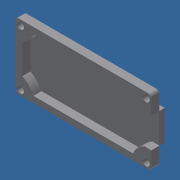
# Autodesk Inventor part: contramoldetapasevo
Saved by Autodesk Inventor 2014 (Build 180170000, 170)
## iProperties
Created: 2014-04-18
Part Number: contramoldetapasevo
Material: Generic
Document SubType Name: Modeling
Designer: Lefo
Density: 1 g/cm^3
Appearance: Default
Author: Lefo
Autodesk Inventor part; units mm, degrees
ref_plane "YZ Plane" through (0, 0, 0) normal (1, 0, 0) x (0, 1, 0)
ref_plane "XZ Plane" through (0, 0, 0) normal (0, 1, 0) x (-1, 0, 0)
sketch "Sketch1" plane through (0, 0, 0) normal (0, 0, 1) x (1, 0, 0)
  line L0 (17.4, 4.3375) -> (19.4, 4.3375) projected
  line L1 (19.4, 8.4) -> (19.4, 4.3375) projected
  arc A0 (19.4, 8.4) -> (18.4, 9.4) centre (18.4, 8.4) ccw projected
  line L2 (-18.4, 9.4) -> (18.4, 9.4) projected
  arc A1 (-18.4, 9.4) -> (-19.4, 8.4) centre (-18.4, 8.4) ccw projected
  line L3 (-19.4, -8.4) -> (-19.4, 8.4) projected
  arc A2 (-19.4, -8.4) -> (-18.4, -9.4) centre (-18.4, -8.4) ccw projected
  line L4 (18.4, -9.4) -> (-18.4, -9.4) projected
  arc A3 (18.4, -9.4) -> (19.4, -8.4) centre (18.4, -8.4) ccw projected
  line L5 (19.4, -4.2375) -> (19.4, -8.4) projected
  line L6 (19.4, -4.2375) -> (17.4, -4.2375) projected
  arc A4 (17.4, -4.2375) -> (14.1485, -7.6) centre (20.15, -10.15) ccw projected
  line L7 (14.1485, -7.6) -> (-14.247, -7.6) projected
  arc A5 (-14.247, -7.6) -> (-17.4, -4.3375) centre (-20.15, -10.15) ccw projected
  line L8 (-17.4, -4.3375) -> (-17.4, 4.2375) projected
  arc A6 (-17.4, 4.2375) -> (-14.1485, 7.6) centre (-20.15, 10.15) ccw projected
  line L9 (-14.1485, 7.6) -> (14.247, 7.6) projected
  arc A7 (14.247, 7.6) -> (17.4, 4.3375) centre (20.15, 10.15) ccw projected
  circle A8 centre (-17.9, -7.9) radius 1 projected
  circle A9 centre (17.9, -7.9) radius 1 projected
  circle A10 centre (-17.9, 7.9) radius 1 projected
  circle A11 centre (17.9, 7.9) radius 1 projected
  line L10 (19.4, -2.5) -> (19.4, 2.5) projected
  line L11 (19.4, 8.4) -> (19.4, 2.5) projected
  line L12 (19.4, -2.5) -> (19.4, -8.4) projected
  point P0 (0, 0)
ref_plane "Work Plane1" through (-26.7016, -22.7609, 2.3) normal (0, 0, 1) x (1, 0, 0)
extrude "Extrusion1" add sketch "Sketch1" along normal up to surface (2.3 mm away) contours A7 L9 A6 L8 A5 L7 A4 L6 L5 A3 L4 A2 L3 A1 L2 A0 L1 L0
sketch "Sketch2" plane through (0, 0, 0) normal (0, 0, -1) x (-1, 0, 0)
  arc A0 (14.1485, 7.6) -> (17.4, 4.2375) centre (20.15, 10.15) ccw projected
  line L0 (17.4, -4.3375) -> (17.4, 4.2375) projected
  arc A1 (17.4, -4.3375) -> (14.247, -7.6) centre (20.15, -10.15) ccw projected
  line L1 (-14.1485, -7.6) -> (14.247, -7.6) projected
  arc A2 (-14.1485, -7.6) -> (-17.4, -4.2375) centre (-20.15, -10.15) ccw projected
  line L2 (-17.4, -4.2375) -> (-19.4, -4.2375) projected
  line L3 (-19.4, -4.2375) -> (-19.4, 4.3375) projected
  line L4 (-19.4, 4.3375) -> (-17.4, 4.3375) projected
  arc A3 (-17.4, 4.3375) -> (-14.247, 7.6) centre (-20.15, 10.15) ccw projected
  line L5 (14.1485, 7.6) -> (-14.247, 7.6) projected
  point P0 (0, 0)
extrude "Extrusion2" add sketch "Sketch2" along normal blind 1.5
sketch "Sketch3" plane through (0, 0, 0) normal (0, 0, 1) x (1, 0, 0)
  line L0 (19.4, 4.3375) -> (19.4, -4.2375) projected
  line L1 (17.4, 4.3375) -> (19.4, 4.3375) projected
  arc A0 (14.247, 7.6) -> (17.4, 4.3375) centre (20.15, 10.15) ccw projected
  line L2 (-14.1485, 7.6) -> (14.247, 7.6) projected
  arc A1 (-17.4, 4.2375) -> (-14.1485, 7.6) centre (-20.15, 10.15) ccw projected
  line L3 (-17.4, -4.3375) -> (-17.4, 4.2375) projected
  arc A2 (-14.247, -7.6) -> (-17.4, -4.3375) centre (-20.15, -10.15) ccw projected
  line L4 (14.1485, -7.6) -> (-14.247, -7.6) projected
  arc A3 (17.4, -4.2375) -> (14.1485, -7.6) centre (20.15, -10.15) ccw projected
  line L5 (19.4, -4.2375) -> (17.4, -4.2375) projected
  arc A4 (13.332, 6.1) -> (17.0815, 2.8375) centre (20.15, 10.15) ccw
  line L6 (17.0815, 2.8375) -> (17.9, 2.8375)
  line L7 (17.9, 2.8375) -> (17.9, -2.7375)
  line L8 (17.9, -2.7375) -> (17.0861, -2.7375)
  arc A5 (17.0861, -2.7375) -> (13.2269, -6.1) centre (20.15, -10.15) ccw
  line L9 (13.2269, -6.1) -> (-13.332, -6.1)
  arc A6 (-13.332, -6.1) -> (-15.9, -3.4548) centre (-20.15, -10.15) ccw
  line L10 (-15.9, -3.4548) -> (-15.9, 3.3478)
  arc A7 (-15.9, 3.3478) -> (-13.2269, 6.1) centre (-20.15, 10.15) ccw
  line L11 (-13.2269, 6.1) -> (13.332, 6.1)
  line L12 (17.9, 2.8375) -> (19.4, 2.8375)
  line L13 (19.4, 2.8375) -> (19.4, -2.7375)
  line L14 (19.4, -2.7375) -> (17.9, -2.7375)
  line L15 (17.9, -2.7375) -> (17.9, 2.8375)
  point P0 (0, 0)
  dimension "d4" = 1.5
  dimension "d5" = 5.575
  constraints: 20 end point, 8 point on circle, 4 centre point, 2 parallel, 1 horizontal, 1 perpendicular, 1 point on line, 9 other
  measures "d4" distance between parallel lines of L2 L11
  measures "d5" distance of L14.end L6.end
extrude "Extrusion3" add sketch "Sketch3" along normal up to surface (2.3 mm away) contours L0 L12 L6 A4 L11 A7 L10 A6 L9 A5 L8 L14 L5 A3 L4 A2 L3 A1 L2 A0 L1
sketch "Sketch4" plane through (-18.4, 9.4, 2.3) normal (0, 0, 1) x (1, 0, 0)
  line L0 (37.8, -12.1375) -> (37.8, -17.8) projected
  line L1 (35.4861, -12.1375) -> (37.8, -12.1375) projected
  arc A0 (35.4861, -12.1375) -> (31.6269, -15.5) centre (38.55, -19.55) ccw projected
  line L2 (5.068, -15.5) -> (31.6269, -15.5) projected
  arc A1 (5.068, -15.5) -> (2.5, -12.8548) centre (-1.75, -19.55) ccw projected
  line L3 (2.5, -6.0522) -> (2.5, -12.8548) projected
  arc A2 (2.5, -6.0522) -> (5.1731, -3.3) centre (-1.75, 0.75) ccw projected
  line L4 (31.732, -3.3) -> (5.1731, -3.3) projected
  arc A3 (31.732, -3.3) -> (35.4815, -6.5625) centre (38.55, 0.75) ccw projected
  line L5 (37.8, -6.5625) -> (35.4815, -6.5625) projected
  line L6 (37.8, -1) -> (37.8, -6.5625) projected
  arc A4 (37.8, -1) -> (36.8, 0) centre (36.8, -1) ccw projected
  line L7 (0, 0) -> (36.8, 0) projected
  arc A5 (0, 0) -> (-1, -1) centre (0, -1) ccw projected
  line L8 (-1, -17.8) -> (-1, -1) projected
  arc A6 (-1, -17.8) -> (0, -18.8) centre (0, -17.8) ccw projected
  line L9 (36.8, -18.8) -> (0, -18.8) projected
  arc A7 (36.8, -18.8) -> (37.8, -17.8) centre (36.8, -17.8) ccw projected
  arc A8 (37.45, -1) -> (36.8, -0.35) centre (36.8, -1) ccw
  line L10 (37.45, -1) -> (37.45, -6.2125)
  line L11 (37.45, -6.2125) -> (35.5528, -6.2125)
  arc A9 (31.9342, -2.95) -> (35.5528, -6.2125) centre (38.55, 0.75) ccw
  line L12 (31.9342, -2.95) -> (4.9694, -2.95)
  arc A10 (2.15, -5.8553) -> (4.9694, -2.95) centre (-1.75, 0.75) ccw
  line L13 (2.15, -5.8553) -> (2.15, -13.05)
  arc A11 (4.8658, -15.85) -> (2.15, -13.05) centre (-1.75, -19.55) ccw
  line L14 (4.8658, -15.85) -> (31.8306, -15.85)
  arc A12 (35.5564, -12.4875) -> (31.8306, -15.85) centre (38.55, -19.55) ccw
  line L15 (35.5564, -12.4875) -> (37.45, -12.4875)
  line L16 (37.45, -12.4875) -> (37.45, -17.8)
  arc A13 (36.8, -18.45) -> (37.45, -17.8) centre (36.8, -17.8) ccw
  line L17 (36.8, -18.45) -> (0, -18.45)
  arc A14 (-0.65, -17.8) -> (0, -18.45) centre (0, -17.8) ccw
  line L18 (-0.65, -17.8) -> (-0.65, -1)
  arc A15 (0, -0.35) -> (-0.65, -1) centre (0, -1) ccw
  line L19 (0, -0.35) -> (36.8, -0.35)
  line L20 (37.45, -6.2125) -> (37.45, -12.4875)
  line L21 (37.8, -6.5625) -> (37.8, -12.1375) projected
  line L22 (37.8, -6.2125) -> (37.8, -1)
  arc A16 (37.8, -1) -> (36.8, 0) centre (36.8, -1) ccw
  line L23 (36.8, 0) -> (0, 0)
  arc A17 (0, 0) -> (-1, -1) centre (0, -1) ccw
  line L24 (-1, -1) -> (-1, -17.8)
  arc A18 (-1, -17.8) -> (0, -18.8) centre (0, -17.8) ccw
  line L25 (0, -18.8) -> (36.8, -18.8)
  arc A19 (36.8, -18.8) -> (37.8, -17.8) centre (36.8, -17.8) ccw
  line L26 (37.8, -17.8) -> (37.8, -12.4875)
  line L27 (37.8, -6.2125) -> (37.8, -12.4875)
  line L28 (-1, 0) -> (37.8, 0)
  line L29 (37.8, 0) -> (37.8, -18.8)
  line L30 (37.8, -18.8) -> (-1, -18.8)
  line L31 (-1, -18.8) -> (-1, 0)
  line L32 (-0.65, -0.35) -> (37.45, -0.35)
  line L33 (37.45, -0.35) -> (37.45, -18.45)
  line L34 (37.45, -18.45) -> (-0.65, -18.45)
  line L35 (-0.65, -18.45) -> (-0.65, -0.35)
  point P0 (18.4, -9.4)
  dimension "d8" = 0.35
  dimension "d9" = 0
  constraints: 50 end point, 24 point on circle, 12 centre point, 4 parallel, 2 collinear, 2 horizontal, 2 perpendicular, 2 point on line, 25 other
  measures "d8" distance between parallel lines of L7 L19
  measures "d9" distance between parallel lines of L23 L7
extrude "Extrusion4" cut sketch "Sketch4" against normal up to surface (2.3 mm away) contours L0 A7 L9 A6 L8 A5 L7 A4 L6 L5 L20 L10 L33 L32 L19 L35 L18 L34 L17 L16 L1 | L20 L15 A12 L14 A11 L13 A10 L12 A9 L11 L5 A3 L4 A2 L3 A1 L2 A0 L1 | L33 L34 A13 | A8 L32 L33 | L34 L35 A14 | A15 L35 L32
body "Solid1"
